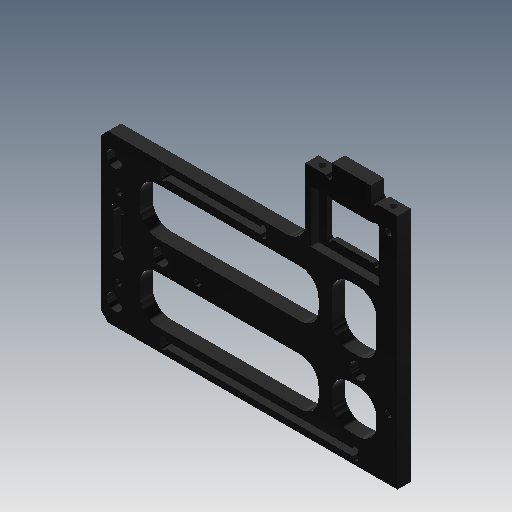
# Autodesk Inventor part: コックピット_2_メインフレーム_1
Saved by Autodesk Inventor 2017.3 (Build 213256000, 256)
## iProperties
Created: 2016-05-24
Part Number: コックピット_2_メインフレーム_1
Material: アセタール樹脂、黒
Document SubType Name: Modeling
Designer: hiroaki
Density: 1.425 g/cm^3
Appearance: 滑らか - 黒
Mass: 29.6333 g
Surface Area: 154.113 cm^2
Volume: 20.7953 cm^3
d0: 1.000 ul
d1: 0.050 mm
d2: 2.100 mm
d3: 2.100 mm
d4: 0.050 mm
d5: 0.050 mm
d6: 5.000 mm
d7: 0.00 deg
d8: 26.000 mm
d9: 20.000 mm
d10: 3.000 mm
d11: 0.00 deg
d12: 27.000 mm
d13: 35.000 mm
d14: 4.000 mm
d16: 2.500 mm
d20: 2.500 mm
d22: 6.000 mm
d23: 5.000 mm
d24: 8.000 mm
d25: 5.000 mm
d26: 5.000 mm
d27: 5.000 mm
d28: 4.000 mm
d29: 0.050 mm
d30: 5.000 mm
d31: 10.000 mm
d32: 0.00 deg
d33: 7.000 mm
d34: 2.400 mm
d35: 7.000 mm
d36: 7.000 mm
d37: 60.000 mm
Author: hiroaki
Autodesk Inventor part; units mm, degrees
ref_plane "YZ Plane" through (0, 0, 0) normal (1, 0, 0) x (0, 1, 0)
ref_plane "XZ Plane" through (0, 0, 0) normal (0, 1, 0) x (-1, 0, 0)
ref_plane "XY Plane" through (0, 0, 0) normal (0, 0, 1) x (1, 0, 0)
derived "コックピット_2_基礎_1.ipt"
sketch "スケッチ1" plane through (0, 0, 0) normal (0, 0, 1) x (1, 0, 0)
  line L0 (47.5, 63.5) -> (62.5, 63.5)
  line L1 (62.5, 63.5) -> (62.5, 58.5)
  line L2 (47.5, 63.5) -> (47.5, 58.5)
  line L3 (64.6, 58.5) -> (72.5, 58.5)
  line L4 (72.5, 58.5) -> (72.5, -31.5)
  line L5 (72.5, -31.5) -> (-37.5, -31.5)
  line L6 (-37.5, -31.5) -> (-37.5, 31.5) construction
  line L7 (-37.5, 31.5) -> (37.5, 31.5)
  line L8 (37.5, 31.5) -> (37.5, 58.5)
  line L9 (37.5, 58.5) -> (45.4, 58.5)
  arc A0 (45.4, 58.5) -> (47.5, 58.5) centre (46.45, 58.5) ccw
  arc A1 (62.5, 58.5) -> (64.6, 58.5) centre (63.55, 58.5) ccw
  circle A2 centre (-17.5, 0) radius 1.55
  circle A3 centre (57.5, 0) radius 1.55
  line L10 (-37.5, 31.5) -> (-32.5, 31.5) construction
  line L11 (-32.5, 31.5) -> (-32.5, -31.5) construction
  line L12 (-32.5, -31.5) -> (-37.5, -31.5) construction
  line L13 (-37.5, -31.5) -> (-37.5, 31.5) construction
  circle A4 centre (-35, 23.5) radius 1.55
  line L14 (-32.5, 2.5) -> (72.5, 2.5) construction
  line L15 (72.5, 2.5) -> (72.5, -2.5) construction
  line L16 (72.5, -2.5) -> (-32.5, -2.5) construction
  line L17 (-32.5, -2.5) -> (-32.5, 2.5) construction
  line L18 (-32.5, -31.5) -> (72.5, -31.5) construction
  line L19 (72.5, -31.5) -> (72.5, -26.5) construction
  line L20 (72.5, -26.5) -> (-32.5, -26.5) construction
  line L21 (-32.5, -26.5) -> (-32.5, -31.5) construction
  line L22 (-32.5, 31.5) -> (37.5, 31.5) construction
  line L23 (37.5, 31.5) -> (37.5, 26.5) construction
  line L24 (37.5, 26.5) -> (-32.5, 26.5) construction
  line L25 (-32.5, 26.5) -> (-32.5, 31.5) construction
  line L26 (-32.5, 8.5) -> (-35, 8.5) construction
  line L27 (-35, 8.5) -> (-35, -8.5) construction
  line L28 (-35, -8.5) -> (-32.5, -8.5) construction
  line L29 (-32.5, -8.5) -> (-32.5, 8.5) construction
  circle A5 centre (-35, -23.5) radius 1.55
  line L30 (-37.5, 0) -> (-53.9458, 0) construction
  line L31 (-37.5, 31.5) -> (-40, 29)
  line L32 (-40, 29) -> (-40, -29)
  line L33 (-40, -29) -> (-37.5, -31.5)
  line L34 (-17.5, -26.5) -> (57.5, -26.5) construction
  line L35 (57.5, -26.5) -> (57.5, -29) construction
  line L36 (57.5, -29) -> (-17.5, -29) construction
  line L37 (-17.5, -29) -> (-17.5, -26.5) construction
  line L38 (-17.5, 26.5) -> (22.5, 26.5) construction
  line L39 (22.5, 26.5) -> (22.5, 29) construction
  line L40 (22.5, 29) -> (-17.5, 29) construction
  line L41 (-17.5, 29) -> (-17.5, 26.5) construction
  circle A6 centre (-35, 23.5) radius 3 construction
  line L42 (42.7, 48.5) -> (62.3, 48.5)
  line L43 (62.3, 48.5) -> (62.3, 35.4)
  line L44 (62.3, 35.4) -> (42.7, 35.4)
  line L45 (42.7, 35.4) -> (42.7, 48.5)
  line L46 (-25.5, 23.5) -> (42.5, 23.5)
  line L47 (42.5, 23.5) -> (42.5, 5.5)
  line L48 (42.5, 5.5) -> (-25.5, 5.5)
  line L49 (-25.5, 5.5) -> (-25.5, 23.5)
  line L50 (-25.5, -5.5) -> (42.5, -5.5)
  line L51 (42.5, -5.5) -> (42.5, -23.5)
  line L52 (42.5, -23.5) -> (-25.5, -23.5)
  line L53 (-25.5, -23.5) -> (-25.5, -5.5)
  circle A7 centre (-17.5, 0) radius 3 construction
  line L54 (-35.05, 8.55) -> (-32.45, 8.55)
  line L55 (-32.45, 8.55) -> (-32.45, -8.55)
  line L56 (-32.45, -8.55) -> (-35.05, -8.55)
  line L57 (-35.05, -8.55) -> (-35.05, 8.55)
  circle A8 centre (-35.05, 7.5) radius 1.05
  circle A9 centre (-32.45, 7.5) radius 1.05
  circle A10 centre (-35.05, -7.5) radius 1.05
  circle A11 centre (-32.45, -7.5) radius 1.05
  line L58 (-17.55, -26.45) -> (57.55, -26.45)
  line L59 (57.55, -26.45) -> (57.55, -29.05)
  line L60 (57.55, -29.05) -> (-17.55, -29.05)
  line L61 (-17.55, -29.05) -> (-17.55, -26.45)
  circle A12 centre (-16.5, -26.45) radius 1.05
  circle A13 centre (-16.5, -29.05) radius 1.05
  circle A14 centre (56.5, -26.45) radius 1.05
  circle A15 centre (56.5, -29.05) radius 1.05
  circle A16 centre (43.75, 48.5) radius 1.05
  circle A17 centre (61.25, 48.5) radius 1.05
  circle A18 centre (61.25, 35.4) radius 1.05
  circle A19 centre (43.75, 35.4) radius 1.05
  line L62 (-17.55, 29.05) -> (22.55, 29.05)
  line L63 (22.55, 29.05) -> (22.55, 26.45)
  line L64 (22.55, 26.45) -> (-17.55, 26.45)
  line L65 (-17.55, 26.45) -> (-17.55, 29.05)
  circle A20 centre (-16.5, 29.05) radius 1.05
  circle A21 centre (-16.5, 26.45) radius 1.05
  circle A22 centre (21.5, 29.05) radius 1.05
  circle A23 centre (21.5, 26.45) radius 1.05
  circle A24 centre (-33.5, -16.5) radius 1.2
  circle A25 centre (-3.5, -1.5) radius 1.2
  circle A26 centre (-33.5, 13.5) radius 1.2
  line L66 (-24.5, -23.5) -> (33.5, -23.5) construction
  line L67 (-22, -23.5) -> (28, -23.5) construction
  line L68 (28, -23.5) -> (28, -16.5) construction
  line L69 (28, -16.5) -> (-22, -16.5) construction
  line L70 (-22, -16.5) -> (-22, -23.5) construction
  circle A27 centre (69, 51.5) radius 1.2
  circle A28 centre (69, 51.5) radius 3.5 construction
  circle A29 centre (69, -8.5) radius 1.2
  point P0 (0, 0)
  point P1 (0, 31.5)
  point P2 (-35, 31.5)
  point P3 (-40, 0)
  point P4 (-32.5, -29)
  point P5 (-32.5, 29)
  point P6 (52.5, 48.5)
  point P7 (55, 63.5)
  dimension "d2" = 2.1
  dimension "d3" = 2.1
  dimension "d1" = 0.05
  dimension "d4" = 0.05
  dimension "d5" = 0.05
  dimension "d34" = 2.4
  dimension "d35" = 7
  dimension "d36" = 7
  dimension "d37" = 60
  measures "d1" distance between parallel lines of L54 L26
  measures "d4" distance between parallel lines of L58 L34
  measures "d5" distance between parallel lines of L62 L40
  measures "d34" diameter of A27
  measures "d35" diameter of A28
  measures "d36" distance from line of L3 A27.centre
  measures "d37" distance of A29.centre A27.centre
extrude "押し出し1" add sketch "スケッチ1" along normal blind 5
sketch "スケッチ3" plane through (-37.5, -31.5, 5) normal (0, 0, 1) x (1, 0, 0)
  line L0 (97.7, 66.9) -> (82.3, 66.9) projected
  arc A0 (80.2, 66.9) -> (82.3, 66.9) centre (81.25, 66.9) ccw projected
  line L1 (80.2, 66.9) -> (80.2, 80) projected
  arc A1 (82.3, 80) -> (80.2, 80) centre (81.25, 80) ccw projected
  line L2 (82.3, 80) -> (97.7, 80) projected
  arc A2 (99.8, 80) -> (97.7, 80) centre (98.75, 80) ccw projected
  line L3 (99.8, 80) -> (99.8, 66.9) projected
  arc A3 (97.7, 66.9) -> (99.8, 66.9) centre (98.75, 66.9) ccw projected
  line L4 (103, 83.45) -> (77, 83.45)
  line L5 (77, 83.45) -> (77, 63.45)
  line L6 (77, 63.45) -> (103, 63.45)
  line L7 (103, 63.45) -> (103, 83.45)
  circle A4 centre (95, 31.5) radius 1.55 projected
  circle A5 centre (20, 31.5) radius 1.55 projected
  circle A6 centre (20, 31.5) radius 3
  circle A7 centre (95, 31.5) radius 3
  circle A8 centre (2.5, 8) radius 1.55 projected
  circle A9 centre (2.5, 55) radius 1.55 projected
  circle A10 centre (2.5, 55) radius 3
  circle A11 centre (2.5, 8) radius 3
  point P0 (37.5, 31.5)
  point P1 (90, 63.45)
  point P2 (90, 66.9)
  point P3 (103, 73.45)
  point P4 (99.8, 73.45)
  dimension "d8" = 26
  dimension "d9" = 20
  dimension "d22" = 6
  constraints: 8 end point, 4 centre point, 4 coincident, 4 midpoint, 3 equal radius, 2 parallel, 1 horizontal, 1 horizontal alignment, 1 perpendicular, 1 vertical alignment
  measures "d8" distance of L5.end L6.end
  measures "d9" distance of L6.end L4.start
  measures "d22" diameter of A6
extrude "押し出し2" cut sketch "スケッチ3" against normal blind 3
sketch "スケッチ4" plane through (37.5, 58.5, 0) normal (0, 1, 0) x (1, 0, 0)
  line L0 (0, 0) -> (0, -5) projected
  line L1 (35, 0) -> (35, -5) projected
  point P0 (-37.5, 0)
  point P1 (4, -2.5)
  point P2 (31, -2.5)
  point P3 (0, -2.5)
  dimension "d12" = 27
  dimension "d13" = 35
  dimension "d14" = 4
  constraints: 2 horizontal alignment, 1 midpoint
  measures "d12" distance of point (31, -2.5) point (4, -2.5)
  measures "d13" distance between parallel lines of L1 L0
  measures "d14" distance from line of L0 point (4, -2.5)
hole "穴1" at (41.5, 58.5, 2.5) at (68.5, 58.5, 2.5) direction (0, -1, 0) diameter 2.459 depth 2.5 thread size "M3x0.5" class "6H" standard "ISO Metric profile"
sketch "スケッチ5" plane through (-37.5, -31.5, 5) normal (0, 0, 1) x (1, 0, 0)
  line L0 (103, 63.45) -> (77, 63.45) projected
  circle A0 centre (95, 31.5) radius 3 projected
  line L1 (80, 55) -> (80, 37) projected
  line L2 (80, 26) -> (80, 8) projected
  line L3 (92.95, 2.45) -> (22.05, 2.45) projected
  arc A1 (19.95, 2.45) -> (22.05, 2.45) centre (21, 2.45) ccw projected
  line L4 (19.95, 2.45) -> (19.95, 5.05) projected
  arc A2 (22.05, 5.05) -> (19.95, 5.05) centre (21, 5.05) ccw projected
  line L5 (22.05, 5.05) -> (92.95, 5.05) projected
  arc A3 (95.05, 5.05) -> (92.95, 5.05) centre (94, 5.05) ccw projected
  line L6 (95.05, 5.05) -> (95.05, 2.45) projected
  arc A4 (92.95, 2.45) -> (95.05, 2.45) centre (94, 2.45) ccw projected
  line L7 (110, 0) -> (110, 90) projected
  line L8 (85, 59.45) -> (102, 59.45)
  line L9 (102, 59.45) -> (102, 36.5)
  line L10 (102, 36.5) -> (85, 36.5)
  line L11 (85, 36.5) -> (85, 59.45)
  line L12 (85, 26.5) -> (102, 26.5)
  line L13 (102, 26.5) -> (102, 10)
  line L14 (102, 10) -> (85, 10)
  line L15 (85, 10) -> (85, 26.5)
  line L16 (93.0013, 5) -> (21.9987, 5)
  arc A5 (21.9987, 5) -> (20, 5.05) centre (21, 5.05) ccw
  line L17 (20, 5.05) -> (20, 2.45)
  arc A6 (20, 2.45) -> (21.9987, 2.5) centre (21, 2.45) ccw
  line L18 (21.9987, 2.5) -> (93.0013, 2.5)
  arc A7 (93.0013, 2.5) -> (95, 2.45) centre (94, 2.45) ccw
  line L19 (95, 2.45) -> (95, 5.05)
  arc A8 (95, 5.05) -> (93.0013, 5) centre (94, 5.05) ccw
  point P0 (37.5, 31.5)
  dimension "d23" = 5
  dimension "d24" = 8
  dimension "d25" = 5
  dimension "d26" = 5
  dimension "d27" = 5
  dimension "d28" = 4
  dimension "d29" = 0.05
  dimension "d30" = 5
  constraints: 24 end point, 8 point on circle, 4 centre point, 4 parallel, 2 horizontal, 2 perpendicular, 1 vertical alignment, 7 other
  measures "d23" distance between parallel lines of L11 L1
  measures "d24" distance between parallel lines of L7 L9
  measures "d25" distance from line of A0.centre L10
  measures "d26" distance from line of L12 A0.centre
  measures "d27" distance between parallel lines of L2 L15
  measures "d28" distance between parallel lines of L0 L8
  measures "d29" distance between parallel lines of L5 L16
  measures "d30" distance between parallel lines of L14 L16
extrude "押し出し3" cut sketch "スケッチ5" against normal blind 10 contours L8 L9 L10 L11 | L12 L13 L14 L15
fillet "フィレット1" radius 7 17 edges at (47.5, 5, 2.5) (42.5, 5.5, 2.5) (47.5, -5, 2.5) (42.5, -5.5, 2.5) (64.5, -5, 2.5) (64.5, 5, 2.5) (64.5, 27.95, 2.5) (47.5, 27.95, 2.5) (42.5, 23.5, 2.5) (-25.5, 23.5, 2.5) (-25.5, 5.5, 2.5) (-25.5, -5.5, 2.5) (-25.5, -23.5, 2.5) (42.5, -23.5, 2.5) (47.5, -21.5, 2.5) (64.5, -21.5, 2.5) (37.5, 31.5, 2.5)
equation "\"d14\" = -0.5 * d12 + 0.5 * d13"
equation "\"d26\" = d25"
equation "\"d27\" = d23"
